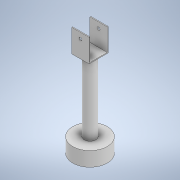
# Autodesk Inventor part: Base Arm 2
Saved by Autodesk Inventor 2020 (Build 240168000, 168)
## iProperties
Created: 2022-02-15
Part Number: Base Arm 2
Material: Generic
Document SubType Name: Modeling
Designer: New-Computer
Density: 1 g/cm^3
Appearance: Default
Mass: 2015.86 g
Surface Area: 1456.23 cm^2
Volume: 2015.86 cm^3
Author: New-Computer
Autodesk Inventor part; units mm, degrees
ref_plane "YZ Plane" through (0, 0, 0) normal (1, 0, 0) x (0, 1, 0)
ref_plane "XZ Plane" through (0, 0, 0) normal (0, 1, 0) x (-1, 0, 0)
ref_plane "XY Plane" through (0, 0, 0) normal (0, 0, 1) x (1, 0, 0)
sketch "Sketch1" plane through (0, 0, 0) normal (0, 1, 0) x (-1, 0, 0)
  circle A0 centre (0, 0) radius 60
  dimension "d0" = 120
  constraints: 1 centre point, 1 coincident
  measures "d0" diameter of A0
extrude "Extrusion1" add sketch "Sketch1" along normal blind 50
sketch "Sketch2" plane through (0, 50, 0) normal (0, 1, 0) x (1, 0, 0)
  circle A0 centre (0, 0) radius 20
  dimension "d3" = 40
  constraints: 1 centre point, 1 coincident
  measures "d3" diameter of A0
extrude "Extrusion2" add sketch "Sketch2" along normal blind 250
sketch "Sketch4" plane through (0, 0, 0) normal (0, -1, 0) x (1, 0, 0)
  circle A0 centre (0, 0) radius 60 projected
  circle A1 centre (0, 0) radius 40.1
  dimension "d11" = 80.2
  constraints: 1 centre point, 1 coincident
  measures "d11" diameter of A1
extrude "Extrusion4" cut sketch "Sketch4" against normal blind 30 contours A1
sketch "Sketch5" plane through (0, 0, 0) normal (0, -1, 0) x (1, 0, 0)
  circle A0 centre (0, 0) radius 20
  dimension "d14" = 40
  constraints: 1 centre point, 1 coincident
  measures "d14" diameter of A0
extrude "Extrusion5" cut sketch "Sketch5" against normal blind 50
sketch "Sketch11" plane through (0, 0, 0) normal (1, 0, 0) x (0, 1, 0)
  line L0 (300, -20) -> (300, 20) projected
  line L1 (300, 33) -> (380, 33)
  line L2 (380, -33) -> (300, -33)
  line L3 (300, -33) -> (300, 33)
  line L4 (300, 0) -> (400, 0)
  line L5 (380, 30) -> (303, 30)
  line L6 (303, 30) -> (303, -30)
  line L7 (303, -30) -> (380, -30)
  line L8 (380, 33) -> (380, 30)
  line L9 (380, -30) -> (380, -33)
  point P0 (0, 0)
  dimension "d50" = 3
  dimension "d51" = 80
  dimension "d52" = 3
  dimension "d64" = 60
  constraints: 18 end point, 5 perpendicular, 4 parallel, 2 horizontal, 2 midpoint, 1 coincident, 3 other
  measures "d50" distance between parallel lines of L1 L5
  measures "d51" distance between parallel lines of L3 L8
  measures "d52" distance between parallel lines of L0 L6
  measures "d64" distance between parallel lines of L7 L5
extrude "Extrusion8" add sketch "Sketch11" along normal mid plane 60
sketch "Sketch12" plane through (30, 380, -33) normal (0, 0, -1) x (-1, 0, 0)
  line L0 (60, -80) -> (0, -80) projected
  line L1 (0, -80) -> (0, 0) projected
  point P0 (30, -380)
  point P1 (30, -20)
  dimension "d55" = 60
  dimension "d56" = 30
  measures "d55" distance from line of point (30, -20) L0
  measures "d56" distance from line of L1 point (30, -20)
hole "Hole3" at (0, 360, -33) direction (0, 0, 1) diameter 10 end through all
body "Solid1"
